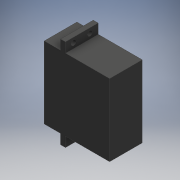
# Autodesk Inventor part: Elbow Servo
Saved by Autodesk Inventor 2017 (Build 210142000, 142)
## iProperties
Created: 2018-10-18
Part Number: Elbow Servo
Material: Generic
Document SubType Name: Modeling
Designer: Cameron
Density: 1 g/cm^3
Appearance: Generic
Author: Cameron
Autodesk Inventor part; units mm, degrees
ref_plane "YZ Plane" through (0, 0, 0) normal (1, 0, 0) x (0, 1, 0)
ref_plane "XZ Plane" through (0, 0, 0) normal (0, 1, 0) x (-1, 0, 0)
ref_plane "XY Plane" through (0, 0, 0) normal (0, 0, 1) x (1, 0, 0)
sketch "Sketch1" plane through (0, 0, 0) normal (0, 1, 0) x (-1, 0, 0)
  line L0 (40, 5) -> (40, -39)
  line L1 (0, -39) -> (0, 0)
  line L2 (40, 5) -> (30, 5)
  line L3 (30, 5) -> (30, 11)
  line L4 (30, 11) -> (27, 11)
  line L5 (27, 11) -> (27, 7)
  line L6 (27, -39) -> (27, -45)
  line L7 (27, -45) -> (30, -45)
  line L8 (30, -45) -> (30, -39)
  line L9 (30, 5) -> (40, 5)
  line L10 (40, -39) -> (30, -39)
  line L11 (27, -39) -> (0, -39)
  line L12 (0, 3) -> (0, 0)
  line L13 (0, 5) -> (0, 3)
  line L14 (27, 5) -> (0, 5)
  line L15 (27, 7) -> (27, 5)
  dimension "d0" = 40
  dimension "d1" = 44
  dimension "d2" = 10
  dimension "d3" = 6
  dimension "d4" = 3
  dimension "d5" = 6
  constraints: 32 end point, 6 perpendicular, 4 point on line, 3 parallel, 1 horizontal
  measures "d0" distance of L0.end L1.start
  measures "d1" distance of L0.start L0.end
  measures "d2" distance of L0.start L2.end
  measures "d3" distance of L2.end L3.end
  measures "d4" distance of L3.end L4.end
  measures "d5" distance of L6.start L6.end
extrude "Extrusion1" add sketch "Sketch1" along normal blind 20
sketch "Sketch2" plane through (-30, 0, 5) normal (-1, 0, 0) x (0, 0, 1)
  line L0 (6, 0) -> (6, 20) projected
  line L1 (6, 10) -> (3, 10)
  line L2 (3, 10) -> (3, 15)
  line L3 (3, 15) -> (3, 5)
  circle A0 centre (3, 15) radius 1.5
  circle A1 centre (3, 5) radius 1.5
  circle A2 centre (-42, 15) radius 1.5
  circle A3 centre (-42, 5) radius 1.5
  dimension "d8" = 5
  dimension "d9" = 10
  dimension "d10" = 3
  dimension "d11" = 3
  dimension "d12" = 3
  dimension "d13" = 3
  constraints: 6 end point, 4 centre point, 2 coincident, 1 horizontal, 1 midpoint, 1 perpendicular, 1 point on line
  measures "d8" distance of L1.end L2.end
  measures "d9" distance of L2.end L3.end
  measures "d10" diameter of A0
  measures "d11" diameter of A1
  measures "d12" diameter of A2
  measures "d13" diameter of A3
extrude "Extrusion2" cut sketch "Sketch2" against normal blind 20
sketch "Sketch3" plane through (-40, 0, -39) normal (-1, 0, 0) x (0, 0, 1)
  line L0 (0, 0) -> (0, 20) projected
  line L1 (0, 10) -> (10, 10)
  circle A0 centre (10, 10) radius 3
  dimension "d16" = 10
  dimension "d17" = 6
  constraints: 2 end point, 1 centre point, 1 coincident, 1 horizontal, 1 midpoint
  measures "d16" distance of L1.start L1.end
  measures "d17" diameter of A0
extrude "Extrusion3" add sketch "Sketch3" along normal blind 4
sketch "Sketch4" plane through (0, 0, 0) normal (1, 0, 0) x (0, 0, -1)
  line L0 (-5, 0) -> (39, 0) projected
  line L1 (39, 0) -> (39, 20) projected
  line L2 (-5, 20) -> (39, 20) projected
  line L3 (0, 0) -> (0, 20) projected
extrude "Extrusion4" cut sketch "Sketch4" against normal blind 2
sketch "Sketch5" plane through (0, 0, 0) normal (0, -1, 0) x (1, 0, 0)
  line L0 (-2, 0) -> (0, 0)
  line L1 (0, 0) -> (0, -39)
  line L2 (0, -39) -> (-2, -39)
  line L3 (-2, -39) -> (-2, 0)
  constraints: 8 end point, 2 parallel, 1 horizontal, 1 perpendicular
extrude "Extrusion5" add sketch "Sketch5" against normal up to surface (20 mm away)
body "Solid1"
